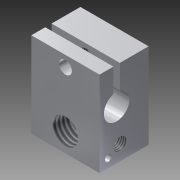
# Autodesk Inventor part: ChimeraHeatBlock
Saved by Autodesk Inventor 2015 SP1 (Build 190203100, 203)
## iProperties
Created: 2014-08-17
Part Number: ChimeraHeatBlock
Material: Aluminum 6061
Document SubType Name: Modeling
Designer: Jack
Density: 2.7 g/cm^3
Appearance: Aluminum - Flat
Author: Jack
Autodesk Inventor part; units mm, degrees
ref_plane "YZ Plane" through (0, 0, 0) normal (1, 0, 0) x (0, 1, 0)
ref_plane "XZ Plane" through (0, 0, 0) normal (0, 1, 0) x (-1, 0, 0)
ref_plane "XY Plane" through (0, 0, 0) normal (0, 0, 1) x (1, 0, 0)
sketch "Sketch1" plane through (0, 0, 0) normal (0, 1, 0) x (-1, 0, 0)
  line L0 (0, 0) -> (16, 0)
  line L1 (16, 0) -> (16, -20)
  line L2 (16, -20) -> (0, -20)
  line L3 (0, -20) -> (0, 0)
  dimension "d0" = 16
  dimension "d1" = 20
  constraints: 8 end point, 2 parallel, 1 horizontal, 1 perpendicular
  measures "d0" distance of L1.end L2.end
  measures "d1" distance of L2.end L0.start
extrude "Extrusion1" add sketch "Sketch1" along normal blind 11.5
sketch "Sketch2" plane through (0, 11.5, 0) normal (0, 1, 0) x (1, 0, 0)
  line L0 (0, 0) -> (0, 20) projected
  line L1 (0, 20) -> (-16, 20) projected
  circle A0 centre (-8, 15.5) radius 3
  dimension "d4" = 6
  dimension "d5" = 8
  dimension "d6" = 4.5
  constraints: 1 centre point
  measures "d4" diameter of A0
  measures "d5" distance from line of L0 A0.centre
  measures "d6" distance from line of L1 A0.centre
extrude "Extrusion2" cut sketch "Sketch2" against normal up to surface (11.5 mm away)
sketch "Sketch3" plane through (0, 11.5, 0) normal (0, 1, 0) x (1, 0, 0)
  line L0 (0, 0) -> (0, 20) projected
  line L1 (0, 20) -> (-16, 20) projected
  circle A0 centre (-8, 2.5) radius 1.5
  dimension "d9" = 3
  dimension "d11" = 17.5
  dimension "d12" = 8
  constraints: 1 centre point
  measures "d9" diameter of A0
  measures "d11" distance from line of L1 A0.centre
  measures "d12" distance from line of L0 A0.centre
extrude "Extrusion3" cut sketch "Sketch3" against normal up to surface (11.5 mm away)
sketch "Sketch4" plane through (0, 0, 0) normal (1, 0, 0) x (0, 0, -1)
  line L0 (20, 0) -> (0, 0) projected
  line L1 (20, 0) -> (20, 11.5) projected
  line L2 (0, 0) -> (0, 11.5) projected
  arc A0 (5.5953, 3.25) -> (5.5953, 4.75) centre (8.5, 4) ccw
  line L3 (5.5953, 4.75) -> (0, 4.75)
  line L4 (5.5953, 3.25) -> (0, 3.25)
  dimension "d15" = 6
  dimension "d16" = 11.5
  dimension "d17" = 4
  dimension "d18" = 1.5
  dimension "d19" = 0.75
  constraints: 4 end point, 2 perpendicular, 2 point on circle, 2 point on line, 1 centre point
  measures "d15" diameter of A0
  measures "d16" distance from line of L1 A0.centre
  measures "d17" distance from line of L0 A0.centre
  measures "d18" distance between parallel lines of L4 L3
  measures "d19" distance from line of A0.centre L3
extrude "Extrusion4" cut sketch "Sketch4" against normal up to surface (16 mm away)
sketch "Sketch5" plane through (0, 0, 0) normal (1, 0, 0) x (0, 0, -1)
  line L0 (20, 0) -> (0, 0) projected
  line L1 (20, 0) -> (20, 11.5) projected
  circle A0 centre (18, 2) radius 0.75
  dimension "d22" = 1.5
  dimension "d24" = 2
  dimension "d25" = 2
  constraints: 1 centre point
  measures "d22" diameter of A0
  measures "d24" distance from line of L0 A0.centre
  measures "d25" distance from line of L1 A0.centre
extrude "Extrusion5" cut sketch "Sketch5" against normal blind 4.4
sketch "Sketch6" plane through (0, 0, 0) normal (1, 0, 0) x (0, 0, -1)
  line L0 (20, 0) -> (0, 0) projected
  line L1 (20, 0) -> (20, 11.5) projected
  circle A0 centre (16.5, 4.8) radius 1.5
  dimension "d28" = 3
  dimension "d29" = 4.8
  dimension "d30" = 3.5
  constraints: 1 centre point
  measures "d28" diameter of A0
  measures "d29" distance from line of L0 A0.centre
  measures "d30" distance from line of L1 A0.centre
extrude "Extrusion6" cut sketch "Sketch6" against normal blind 3.4
thread "Thread1" size "M3x0.5" class "6H" standard "ANSI Metric M Profile" full length
thread "Thread2" size "M6x1" class "6H" standard "ANSI Metric M Profile" full length
thread "Thread3" size "M3x0.5" class "6H" standard "ANSI Metric M Profile" full length
body "Solid1"
